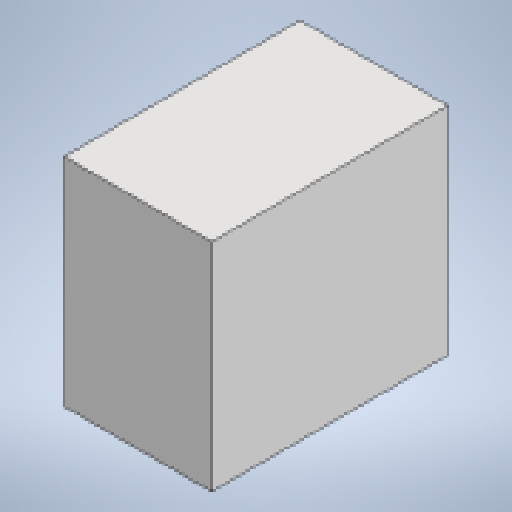
# Autodesk Inventor part: NDM-VOS dummy staircase
Saved by Autodesk Inventor 2025 (Build 290162010, 162A)
## iProperties
Created: 2024-10-13
Part Number: NDM-VOS dummy staircase
Material: Generic
Document SubType Name: Modeling
Designer: admin
Density: 1 g/cm^3
Appearance: Default
Author: admin
Autodesk Inventor part; units mm, degrees
ref_plane "YZ Plane" through (0, 0, 0) normal (1, 0, 0) x (0, 1, 0)
ref_plane "XZ Plane" through (0, 0, 0) normal (0, 1, 0) x (-1, 0, 0)
ref_plane "XY Plane" through (0, 0, 0) normal (0, 0, 1) x (1, 0, 0)
sketch "Sketch1" plane through (0, 0, 0) normal (0, 0, 1) x (1, 0, 0)
  line L0 (-750, 1300) -> (750, 1300)
  line L1 (750, 1300) -> (750, -1300)
  line L2 (750, -1300) -> (-750, -1300)
  line L3 (-750, -1300) -> (-750, 1300)
  line L4 (-750, 1300) -> (750, -1300) construction
  line L5 (750, 1300) -> (-750, -1300) construction
  point P0 (0, 0)
  dimension "d0" = 1500
  dimension "d1" = 2600
  constraints: 12 end point, 2 midpoint, 2 parallel, 1 horizontal, 1 perpendicular
  measures "d0" distance of L1.end L2.end
  measures "d1" distance of L0.end L1.end
extrude "Extrusion1" add sketch "Sketch1" along normal blind 2200
body "Solid1"
